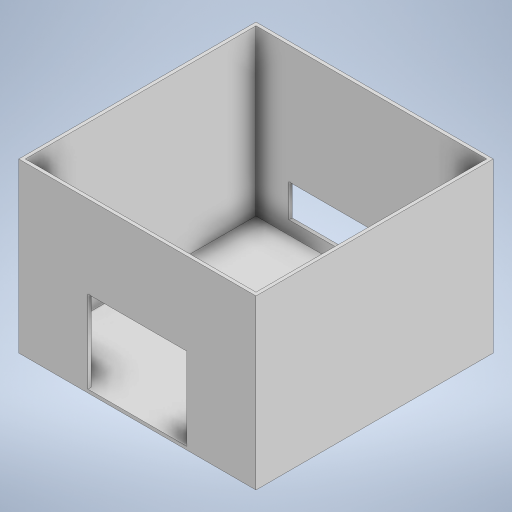
# Autodesk Inventor part: Part2 Zaid
Saved by Autodesk Inventor 2023 (Build 270158030, 158C)
## iProperties
Created: 2023-04-28
Part Number: Part2 Zaid
Material: Generic
Document SubType Name: Modeling
Designer: 22165
Density: 1 g/cm^3
Appearance: Default
Author: 22165
Autodesk Inventor part; units mm, degrees
ref_plane "YZ Plane" through (0, 0, 0) normal (1, 0, 0) x (0, 1, 0)
ref_plane "XZ Plane" through (0, 0, 0) normal (0, 1, 0) x (-1, 0, 0)
ref_plane "XY Plane" through (0, 0, 0) normal (0, 0, 1) x (1, 0, 0)
sketch "Sketch1" plane through (0, 0, 0) normal (0, 0, 1) x (1, 0, 0)
  line L0 (0, 0) -> (140, 0)
  line L1 (140, 0) -> (140, -100)
  line L2 (140, -100) -> (0, -100)
  line L3 (0, -100) -> (0, 0)
  dimension "d0" = 100
  dimension "d1" = 140
  constraints: 8 end point, 2 parallel, 1 horizontal, 1 perpendicular
  measures "d0" distance of L0.end L1.end
  measures "d1" distance of L1.end L2.end
extrude "Extrusion1" add sketch "Sketch1" along normal blind 140
shell "Shell1" thickness 2 outward yes removed faces 1 at (93.3333, 0, 93.3333)
sketch "Sketch2" plane through (0, 0, 142) normal (0, 0, 1) x (1, 0, 0)
  line L0 (0, -100) -> (140, -100) projected
  line L1 (40, -50) -> (100, -50)
  line L2 (100, -50) -> (100, -100)
  line L3 (100, -100) -> (40, -100)
  line L4 (40, -100) -> (40, -50)
  line L5 (0, 0) -> (0, -100) projected
  line L6 (140, -100) -> (140, 0) projected
  line L7 (142, 0) -> (-2, 0) projected
  point P0 (40, -75)
  dimension "d5" = 40
  dimension "d6" = 40
  dimension "d7" = 50
  constraints: 8 end point, 2 parallel, 1 horizontal, 1 midpoint, 1 perpendicular, 1 point on line
  measures "d5" distance from line of L5 point (40, -75)
  measures "d6" distance between parallel lines of L6 L2
  measures "d7" distance between parallel lines of L7 L1
extrude "Extrusion2" cut sketch "Sketch2" against normal blind 14 contours L4 L1 L2 L0
sketch "Sketch3" plane through (0, 0, -2) normal (0, 0, -1) x (-1, 0, 0)
  line L0 (-120, -72) -> (-20, -72)
  line L1 (-20, -72) -> (-20, -92)
  line L2 (-20, -92) -> (-120, -92)
  line L3 (-120, -92) -> (-120, -72)
  line L4 (0, 0) -> (0, -100) projected
  line L5 (-140, -100) -> (-140, 0) projected
  line L6 (2, -102) -> (-142, -102) projected
  point P0 (-120, -82)
  dimension "d13" = 20
  dimension "d14" = 20
  dimension "d15" = 20
  dimension "d16" = 10
  constraints: 8 end point, 2 parallel, 1 horizontal, 1 midpoint, 1 perpendicular
  measures "d13" distance between parallel lines of L2 L0
  measures "d14" distance between parallel lines of L4 L1
  measures "d15" distance from line of L5 point (-120, -82)
  measures "d16" distance between parallel lines of L6 L2
extrude "Extrusion4" cut sketch "Sketch3" against normal blind 10
body "Solid1"
